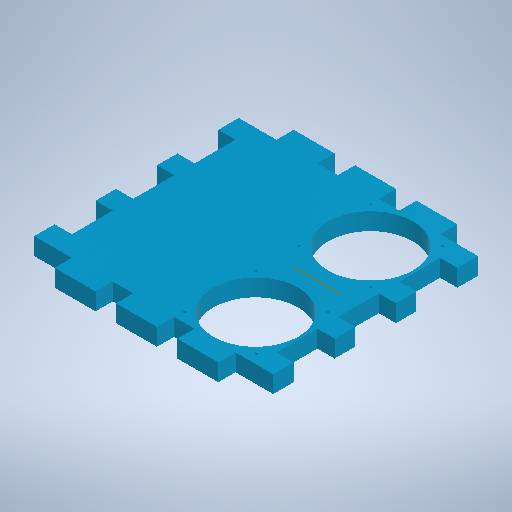
# Autodesk Inventor part: 4
Saved by Autodesk Inventor 2025.3 (Build 293356000, 356)
## iProperties
Created: 2025-12-22
Part Number: 4
Material: Generic
Document SubType Name: Sheet Metal
Designer: Balint
Density: 1 g/cm^3
Flat Pattern Width: 25 cm
Flat Pattern Length: 25 cm
Flat Pattern Area: 625 cm^2
Sheet Metal Rule: Default_mm
Sheet Metal Width: 250.000 mm
Sheet Metal Length: 250.000 mm
Sheet Metal Area: 62500.000 mm^2
Appearance: Sky Blue Dark
Author: Balint
Autodesk Inventor part; units mm, degrees
ref_plane "YZ Plane" through (0, 0, 0) normal (1, 0, 0) x (0, 1, 0)
ref_plane "XZ Plane" through (0, 0, 0) normal (0, 1, 0) x (-1, 0, 0)
ref_plane "XY Plane" through (0, 0, 0) normal (0, 0, 1) x (1, 0, 0)
sketch "Sketch1" plane through (0, 0, 0) normal (0, 1, 0) x (-1, 0, 0)
  line L0 (-127.7724, 127.5062) -> (122.2276, 127.5062)
  line L1 (122.2276, 127.5062) -> (122.2276, -122.4938)
  line L2 (122.2276, -122.4938) -> (-127.7724, -122.4938)
  line L3 (-127.7724, -122.4938) -> (-127.7724, 127.5062)
  line L4 (104.2276, -104.4938) -> (104.2276, 109.5062)
  line L5 (104.2276, -104.4938) -> (-109.7724, -104.4938)
  line L6 (-109.7724, -104.4938) -> (104.2276, -104.4938)
  line L7 (122.2276, 109.5062) -> (122.2276, 88.1062)
  line L8 (122.2276, 88.1062) -> (104.2276, 88.1062)
  line L9 (104.2276, 88.1062) -> (104.2276, 109.5062)
  line L10 (122.2276, 45.3062) -> (104.2276, 45.3062)
  line L11 (104.2276, 45.3062) -> (104.2276, 23.9062)
  line L12 (104.2276, 23.9062) -> (122.2276, 23.9062)
  line L13 (104.2276, -18.8938) -> (122.2276, -18.8938)
  line L14 (122.2276, -40.2938) -> (104.2276, -40.2938)
  line L15 (122.2276, -83.0938) -> (104.2276, -83.0938)
  line L16 (-127.7724, 127.5062) -> (-127.7724, 109.5062)
  line L17 (104.2276, 109.5062) -> (104.2276, 127.5062)
  line L18 (-127.7724, -83.0938) -> (-109.7724, -83.0938)
  line L19 (-127.7724, -40.2938) -> (-109.7724, -40.2938)
  line L20 (-109.7724, -18.8938) -> (-127.7724, -18.8938)
  line L21 (-109.7724, 23.9062) -> (-127.7724, 23.9062)
  line L22 (-127.7724, 45.3062) -> (-109.7724, 45.3062)
  line L23 (-127.7724, 88.1062) -> (-109.7724, 88.1062)
  line L24 (18.6276, -104.4938) -> (18.6276, -122.4938)
  line L25 (-24.1724, -104.4938) -> (-24.1724, -122.4938)
  line L26 (-45.5724, -122.4938) -> (-45.5724, -104.4938)
  line L27 (-88.3724, -122.4938) -> (-88.3724, -104.4938)
  line L28 (40.0276, -122.4938) -> (40.0276, -104.4938)
  line L29 (82.8276, -122.4938) -> (82.8276, -104.4938)
  line L30 (18.6276, 127.5062) -> (18.6276, 109.5062)
  line L31 (40.0276, 109.5062) -> (40.0276, 127.5062)
  line L32 (82.8276, 109.5062) -> (82.8276, 127.5062)
  line L33 (-45.5724, 109.5062) -> (-45.5724, 127.5062)
  line L34 (-88.3724, 109.5062) -> (-88.3724, 127.5062)
  line L35 (-24.1724, 127.5062) -> (-24.1724, 109.5062)
  line L36 (104.2276, 109.5062) -> (-109.7724, 109.5062)
  line L37 (-109.7724, 109.5062) -> (-109.7724, -104.4938)
  line L38 (-109.7724, 109.5062) -> (-127.7724, 109.5062)
  line L39 (-127.7724, 109.5062) -> (-127.7724, 127.5062)
  line L40 (-127.7724, 127.5062) -> (-109.7724, 127.5062)
  line L41 (-109.7724, 127.5062) -> (-109.7724, 109.5062)
  line L42 (-109.7724, -104.4938) -> (-127.7724, -104.4938)
  line L43 (-127.7724, -104.4938) -> (-127.7724, -122.4938)
  line L44 (-127.7724, -122.4938) -> (-109.7724, -122.4938)
  line L45 (-109.7724, -122.4938) -> (-109.7724, -104.4938)
  line L46 (104.2276, -104.4938) -> (122.2276, -104.4938)
  line L47 (122.2276, -104.4938) -> (122.2276, -122.4938)
  line L48 (122.2276, -122.4938) -> (104.2276, -122.4938)
  line L49 (104.2276, -122.4938) -> (104.2276, -104.4938)
  line L50 (104.2276, 109.5062) -> (122.2276, 109.5062)
  line L51 (122.2276, 109.5062) -> (122.2276, 127.5062)
  line L52 (122.2276, 127.5062) -> (104.2276, 127.5062)
  line L53 (104.2276, 127.5062) -> (104.2276, 109.5062)
  point P0 (0, 0)
  point P1 (-127.7724, -18.8938)
  point P2 (-109.7724, -104.4938)
  point P3 (-109.7724, -104.4938)
  dimension "d0" = 250
  dimension "d1" = 250
  dimension "d2" = 21.4
  measures "d0" distance of L1.end L2.end
  measures "d1" distance of L0.end L1.end
  measures "d2" distance of L7.start L7.end
extrude "Plate1" add sketch "Sketch1" along normal blind 18 contours L38 L37 L23 L3 | L0 L33 L36 L34 | L36 L4 L5 L37 | L22 L37 L21 L3 | L0 L30 L36 L35 | L20 L37 L19 L3 | L0 L32 L36 L31 | L18 L37 L42 L3 | L50 L1 L8 L4 | L5 L26 L2 L27 | L10 L1 L12 L4 | L5 L24 L2 L25 | L13 L1 L14 L4 | L5 L29 L2 L28 | L15 L1 L46 L4
sketch "Sketch2" plane through (0, 0, 0) normal (0, -1, 0) x (1, 0, 0)
  line L0 (0, 0) -> (125, 0)
  line L1 (125, 0) -> (125, 125)
  line L2 (125, 125) -> (0, 125)
  line L3 (0, 125) -> (0, 0)
  line L4 (125, 125) -> (62.5, 125)
  line L5 (125, 62.5) -> (125, 125)
  circle A0 centre (62.5, 62.5) radius 44.45
  line L6 (25, 100) -> (100, 100)
  line L7 (100, 100) -> (100, 25)
  line L8 (100, 25) -> (25, 25)
  line L9 (25, 25) -> (25, 100)
  line L10 (25, 100) -> (100, 25) construction
  line L11 (100, 100) -> (25, 25) construction
  circle A1 centre (100, 100) radius 1.5
  circle A2 centre (100, 25) radius 1.5
  circle A3 centre (25, 25) radius 1.5
  circle A4 centre (25, 100) radius 1.5
  dimension "d4" = 125
  dimension "d5" = 125
  dimension "d6" = 88.9
  dimension "d7" = 75
  dimension "d8" = 75
  dimension "d9" = 3
  dimension "d10" = 3
  dimension "d11" = 3
  dimension "d12" = 3
  constraints: 24 end point, 5 centre point, 4 coincident, 4 parallel, 3 horizontal, 2 midpoint, 2 perpendicular
  measures "d4" distance of L2.end L1.end
  measures "d5" distance of L1.end L0.end
  measures "d6" diameter of A0
  measures "d7" distance of L7.end L8.end
  measures "d8" distance of L6.end L7.end
  measures "d9" diameter of A1
  measures "d10" diameter of A2
  measures "d11" diameter of A3
  measures "d12" diameter of A4
extrude "Cut1" cut sketch "Sketch2" against normal blind 18 contours A0 L7 | L7 A0 L8 L9 L6 | L6 A0 | A1 L6 L7 | L7 L6 A1 | A0 L8 | A2 L8 L7 | L7 L8 A2 | L9 A0 | A4 L9 L6 | L6 L9 A4 | A3 L9 L8 | L8 L9 A3
ref_plane "Work Plane1" through (45.5724, 0, 2.5062) normal (0, 0, 1) x (1, 0, 0)
mirror "Mirror1" about plane through (45.5724, 0, 2.5062) normal (0, 0, 1) of "Cut1"
equation "\"d13\" = Thickness"
equation "\"d3\" = Thickness"
equation "\"BendRadius\" = Thickness"
equation "\"BendReliefWidth\" = Thickness"
equation "\"BendReliefDepth\" = 0.5 * Thickness"
equation "\"CornerReliefSize\" = 4 * Thickness"
equation "\"MinimumRemnant\" = 2 * Thickness"
equation "\"TransitionRadius\" = BendRadius"
equation "\"JacobiRadiusSize\" = BendRadius"
equation "\"GapSize\" = Thickness"
equation "\"Thickness\" = 18"
body "Solid1"
